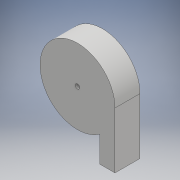
# Autodesk Inventor part: Pump_case
Saved by Autodesk Inventor 2017 (Build 210142000, 142)
## iProperties
Created: 2016-12-23
Part Number: Pump_case
Material: Generic
Document SubType Name: Modeling
Designer: Ali
Density: 1 g/cm^3
Appearance: Default
Author: Ali
Autodesk Inventor part; units mm, degrees
ref_plane "YZ Plane" through (0, 0, 0) normal (1, 0, 0) x (0, 1, 0)
ref_plane "XZ Plane" through (0, 0, 0) normal (0, 1, 0) x (-1, 0, 0)
ref_plane "XY Plane" through (0, 0, 0) normal (0, 0, 1) x (1, 0, 0)
sketch "Sketch1" plane through (0, 0, 0) normal (0, 1, 0) x (-1, 0, 0)
  circle A0 centre (0, 0) radius 25
  circle A1 centre (0, 0) radius 30
  line L0 (-30, 0) -> (-30, -45)
  line L1 (-30, -45) -> (-18, -45)
  line L2 (-18, -45) -> (-18, -24)
  dimension "d0" = 50
  dimension "d1" = 60
  dimension "d4" = 45
  dimension "d5" = 12
  constraints: 6 end point, 2 centre point, 2 coincident, 2 perpendicular, 2 point on circle, 1 tangent, 1 vertical
  measures "d0" diameter of A0
  measures "d1" diameter of A1
  measures "d4" distance of L0.start L0.end
  measures "d5" distance of L0.end L1.end
extrude "Extrusion1" add sketch "Sketch1" along normal blind 20 contours A0 | A1 | A1 L2 L1 L0
shell "Shell1" thickness 3 removed faces 1 at (26, 6.6667, -45)
sketch "Sketch11" plane through (21, 3, -45) normal (0, 1, 0) x (1, 0, 0)
  circle A0 centre (-21, -45) radius 30
  dimension "d44" = 60
  constraints: 1 centre point, 1 coincident
  measures "d44" diameter of A0
extrude "Extrusion9" cut sketch "Sketch11" against normal blind 5
sketch "Sketch12" plane through (21, 3, -45) normal (0, -1, 0) x (1, 0, 0)
  circle A0 centre (-21, 45) radius 30
  constraints: 1 centre point, 1 coincident
extrude "Extrusion10" add sketch "Sketch12" along normal blind 3
sketch "Sketch14" plane through (0, 20, 0) normal (0, 1, 0) x (1, 0, 0)
  circle A0 centre (0, 0) radius 27
  dimension "d57" = 54
  constraints: 1 centre point, 1 coincident
  measures "d57" diameter of A0
extrude "Extrusion11" cut sketch "Sketch14" against normal blind 14
sketch "Sketch13" plane through (21, 3, -45) normal (0, 1, 0) x (1, 0, 0)
  circle A0 centre (-21, -45) radius 1.75
  dimension "d49" = 3.5
  constraints: 1 centre point, 1 coincident
  measures "d49" diameter of A0
hole "Hole3" at (0, 3, 0) direction (0, -1, 0) diameter 3.5 depth 3
body "Solid1"
